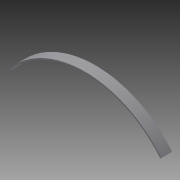
# Autodesk Inventor part: Shooter_3inRollerGuide
Saved by Autodesk Inventor 2014 (Build 180170000, 170)
## iProperties
Created: 2016-01-26
Part Number: Shooter_3inRollerGuide
Material: Generic
Document SubType Name: Modeling
Designer: choices
Density: 1 g/cm^3
Appearance: Default
Author: choices
Autodesk Inventor part; units mm, degrees
ref_plane "YZ Plane" through (0, 0, 0) normal (1, 0, 0) x (0, 1, 0)
ref_plane "XZ Plane" through (0, 0, 0) normal (0, 1, 0) x (-1, 0, 0)
ref_plane "XY Plane" through (0, 0, 0) normal (0, 0, 1) x (1, 0, 0)
sketch "Sketch2" plane through (0, 0, 0) normal (0, 0, 1) x (1, 0, 0)
  line L0 (0, 0) -> (355.6, 0)
  arc A0 (355.6, 0) -> (0, 0) centre (177.8, -143.6841) ccw
  circle A1 centre (177.8, -143.6841) radius 231.775
  line L1 (177.8, -143.6841) -> (0, 0)
  line L2 (177.8, -143.6841) -> (355.6, 0)
  line L3 (355.6, 0) -> (358.0694, 1.9956)
  line L4 (0, 0) -> (-2.4694, 1.9956)
  dimension "d0" = 355.6
  dimension "d2" = 228.6
  dimension "d3" = 463.55
  constraints: 10 end point, 4 point on circle, 2 centre point, 2 collinear, 1 coincident, 1 horizontal
  measures "d0" distance of L0.start L0.end
  measures "d2" radius of A0
  measures "d3" diameter of A1
extrude "Extrusion1" add sketch "Sketch2" along normal blind 25.4 contours L4 A1 L3 A0
body "Solid1"
